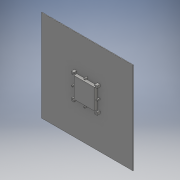
# Autodesk Inventor part: Motor-support_chassis-fit_hold-wheels_spencermical_ENES100-OSV
Saved by Autodesk Inventor 2016 (Build 200138000, 138)
## iProperties
Created: 2016-03-08
Part Number: Motor-support_chassis-fit_hold-wheels_spencermical_ENES100-OSV
Material: Generic
Document SubType Name: Modeling
Designer: Spencer
Density: 1 g/cm^3
Appearance: Default
Author: Spencer
Autodesk Inventor part; units mm, degrees
ref_plane "YZ Plane" through (0, 0, 0) normal (1, 0, 0) x (0, 1, 0)
ref_plane "XZ Plane" through (0, 0, 0) normal (0, 1, 0) x (-1, 0, 0)
ref_plane "XY Plane" through (0, 0, 0) normal (0, 0, 1) x (1, 0, 0)
sketch "Sketch1" plane through (0, 0, 0) normal (0, 1, 0) x (-1, 0, 0)
  line L0 (27.5, 18.707) -> (-27.5, 18.707)
  line L1 (-27.5, 18.707) -> (-27.5, -18.707)
  line L2 (-27.5, -18.707) -> (27.5, -18.707)
  line L3 (27.5, -18.707) -> (27.5, 18.707)
  line L4 (27.5, 18.707) -> (-27.5, -18.707) construction
  line L5 (-27.5, 18.707) -> (27.5, -18.707) construction
  point P0 (0, 0)
  dimension "d0" = 37.414
  dimension "d1" = 55
  constraints: 12 end point, 2 midpoint, 2 parallel, 1 horizontal, 1 perpendicular
  measures "d0" distance of L2.end L0.start
  measures "d1" distance of L1.end L2.end
extrude "Extrusion1" add sketch "Sketch1" along normal blind 30.404
sketch "Sketch2" plane through (0, 30.404, 0) normal (0, 1, 0) x (1, 0, 0)
  line L0 (-26.5, -17.707) -> (26.5, -17.707)
  line L1 (26.5, -17.707) -> (26.5, 17.707)
  line L2 (26.5, 17.707) -> (-26.5, 17.707)
  line L3 (-26.5, 17.707) -> (-26.5, -17.707)
  line L4 (-26.5, -17.707) -> (26.5, 17.707) construction
  line L5 (26.5, -17.707) -> (-26.5, 17.707) construction
  point P0 (0, 0)
  dimension "d4" = 35.414
  dimension "d5" = 53
  constraints: 12 end point, 2 midpoint, 2 parallel, 1 horizontal, 1 perpendicular
  measures "d4" distance of L2.end L0.start
  measures "d5" distance of L1.end L2.end
extrude "Extrusion2" cut sketch "Sketch2" against normal blind 29.404
sketch "Sketch6" plane through (0, 0, 0) normal (0, -1, 0) x (1, 0, 0)
  line L0 (175, 175) -> (-175, 175)
  line L1 (-175, 175) -> (-175, -175)
  line L2 (-175, -175) -> (175, -175)
  line L3 (175, -175) -> (175, 175)
  line L4 (175, 175) -> (-175, -175) construction
  line L5 (-175, 175) -> (175, -175) construction
  point P0 (0, 0)
  dimension "d19" = 350
  dimension "d20" = 350
  constraints: 12 end point, 2 midpoint, 2 parallel, 1 horizontal, 1 perpendicular
  measures "d19" distance of L2.end L0.start
  measures "d20" distance of L1.end L2.end
extrude "Extrusion4" add sketch "Sketch6" along normal blind 2
sketch "Sketch7" plane through (0, -2, 0) normal (0, -1, 0) x (1, 0, 0)
  line L0 (39.5, 39.5) -> (-39.5, 39.5)
  line L1 (-39.5, 39.5) -> (-39.5, -39.5)
  line L2 (-39.5, -39.5) -> (39.5, -39.5)
  line L3 (39.5, -39.5) -> (39.5, 39.5)
  line L4 (39.5, 39.5) -> (-39.5, -39.5) construction
  line L5 (-39.5, 39.5) -> (39.5, -39.5) construction
  point P0 (0, 0)
  dimension "d23" = 79
  dimension "d24" = 79
  constraints: 12 end point, 2 midpoint, 2 parallel, 1 horizontal, 1 perpendicular
  measures "d23" distance of L2.end L0.start
  measures "d24" distance of L0.start L0.end
extrude "Extrusion5" add sketch "Sketch7" along normal blind 11
sketch "Sketch8" plane through (0, -2, 0) normal (0, -1, 0) x (1, 0, 0)
  line L0 (2.3, -49) -> (-2.2, -49)
  line L1 (-2.2, -49) -> (-2.2, -44.5)
  line L2 (-2.2, -44.5) -> (2.3, -44.5)
  line L3 (2.3, -44.5) -> (2.3, -49)
  line L4 (2.3, -49) -> (-2.2, -44.5) construction
  line L5 (-2.2, -49) -> (2.3, -44.5) construction
  line L6 (-39.5, -39.5) -> (39.5, -39.5) projected
  line L7 (-175, 175) -> (-175, -175) projected
  point P0 (0, 0)
  point P1 (0.05, -46.75)
  dimension "d27" = 5
  dimension "d28" = 4.5
  dimension "d29" = 4.5
  dimension "d30" = 172.8
  constraints: 12 end point, 2 midpoint, 2 parallel, 1 horizontal, 1 perpendicular
  measures "d27" distance from line of L1.end L6
  measures "d28" distance of L2.end L0.start
  measures "d29" distance of L0.start L0.end
  measures "d30" distance from line of L7 L0.end
extrude "Extrusion6" add sketch "Sketch8" along normal blind 11
mirror "Mirror1" about plane through (0, 0, 0) normal (0, 0, 1) of "Extrusion6"
sketch "Sketch9" plane through (0, -2, 0) normal (0, -1, 0) x (1, 0, 0)
  line L0 (49, -2.3) -> (44.5, -2.3)
  line L1 (44.5, -2.3) -> (44.5, 2.2)
  line L2 (44.5, 2.2) -> (49, 2.2)
  line L3 (49, 2.2) -> (49, -2.3)
  line L4 (49, -2.3) -> (44.5, 2.2) construction
  line L5 (44.5, -2.3) -> (49, 2.2) construction
  line L6 (39.5, -39.5) -> (39.5, 39.5) projected
  line L7 (175, 175) -> (-175, 175) projected
  point P0 (0, 0)
  point P1 (46.75, -0.05)
  dimension "d33" = 5
  dimension "d34" = 4.5
  dimension "d35" = 4.5
  dimension "d36" = 172.8
  constraints: 12 end point, 2 midpoint, 2 parallel, 1 horizontal, 1 perpendicular
  measures "d33" distance from line of L1.end L6
  measures "d34" distance of L1.end L2.end
  measures "d35" distance of L2.end L0.start
  measures "d36" distance from line of L7 L2.end
extrude "Extrusion7" add sketch "Sketch9" along normal blind 11
mirror "Mirror2" about plane through (0, 0, 0) normal (1, 0, 0) of "Extrusion7"
sketch "Sketch10" plane through (0, -2, 0) normal (0, -1, 0) x (1, 0, 0)
  line L0 (49, 2.2) -> (49, -2.3) projected
  line L1 (49, -2.3) -> (49, -53.869)
  line L2 (2.3, -49) -> (58.6283, -49)
  line L3 (49, -49) -> (44.5, -49)
  line L4 (44.5, -49) -> (44.5, -39.5)
  line L5 (44.5, -39.5) -> (49, -39.5)
  line L6 (49, -39.5) -> (49, -49)
  line L7 (44.5, -44.25) -> (39.5, -44.25)
  line L8 (39.5, -44.25) -> (39.5, -49)
  line L9 (39.5, -49) -> (44.5, -49)
  line L10 (44.5, -49) -> (44.5, -44.25)
  point P0 (0, 0)
  dimension "d39" = 9.5
  dimension "d40" = 4.5
  dimension "d41" = 5
  dimension "d42" = 4.75
  constraints: 20 end point, 4 parallel, 3 horizontal, 3 point on line, 2 perpendicular, 1 midpoint, 1 vertical
  measures "d39" distance of L3.end L4.end
  measures "d40" distance of L4.end L5.end
  measures "d41" distance of L7.start L7.end
  measures "d42" distance of L7.end L8.end
extrude "Extrusion8" add sketch "Sketch10" along normal blind 11
mirror "Mirror3" about plane through (0, 0, 0) normal (0, 0, 1) of "Extrusion8"
mirror "Mirror4" about plane through (0, 0, 0) normal (1, 0, 0) of "Extrusion8", "Mirror3"
body "Solid1"
